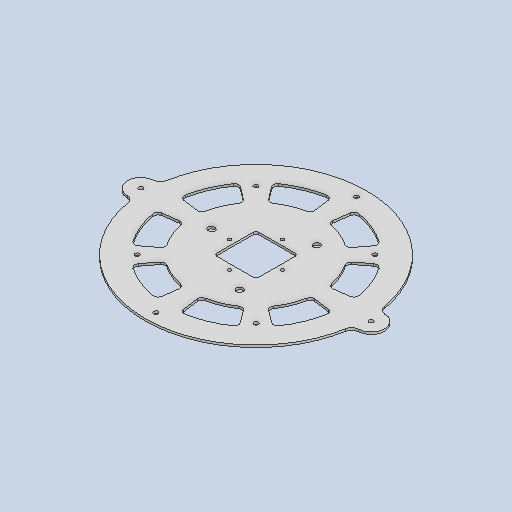
# Autodesk Inventor part: AP-1-02-basePlate
Saved by Autodesk Inventor 2025.1 (Build 291241020, 241B)
## iProperties
Created: 2024-10-16
Part Number: AP-1-02-basePlate
Material: Generic
Document SubType Name: Modeling
Designer: jdl5984
Density: 1 g/cm^3
Appearance: Default
Author: jdl5984
## iProperties of the stored document AP-1-02-basePlate_3DPrint.ipt
Created: 2024-12-05
Part Number: AP-1-02-basePlate_3DPrint
Material: Generic
Document SubType Name: Modeling
Designer: t205b
Density: 1 g/cm^3
Appearance: Default
Author: t205b
Autodesk Inventor part; units mm, degrees
ref_plane "YZ Plane" through (0, 0, 0) normal (1, 0, 0) x (0, 1, 0)
ref_plane "XZ Plane" through (0, 0, 0) normal (0, 1, 0) x (-1, 0, 0)
ref_plane "XY Plane" through (0, 0, 0) normal (0, 0, 1) x (1, 0, 0)
sketch "Sketch1" plane through (0, 0, 0) normal (0, 1, 0) x (-1, 0, 0)
  circle A0 centre (0, 0) radius 158.75
  line L0 (26.05, 30.05) -> (-26.05, 30.05)
  line L1 (-30.05, 26.05) -> (-30.05, -26.05)
  line L2 (-26.05, -30.05) -> (26.05, -30.05)
  line L3 (30.05, -26.05) -> (30.05, 26.05)
  arc A1 (30.05, 26.05) -> (26.05, 30.05) centre (26.05, 26.05) ccw
  arc A2 (26.05, -30.05) -> (30.05, -26.05) centre (26.05, -26.05) ccw
  arc A3 (-30.05, -26.05) -> (-26.05, -30.05) centre (-26.05, -26.05) ccw
  arc A4 (-26.05, 30.05) -> (-30.05, 26.05) centre (-26.05, 26.05) ccw
  circle A5 centre (38, 0) radius 2.5527
  circle A6 centre (0, -38) radius 2.5527
  circle A7 centre (-38, 0) radius 2.5527
  circle A8 centre (0, 38) radius 2.5527
  circle A9 centre (63.9092, 0) radius 4.7625
  circle A10 centre (-31.9546, -55.3454) radius 4.7625
  circle A11 centre (0, 0) radius 63.9092 construction
  circle A12 centre (0, 143.6497) radius 3.2067
  circle A13 centre (0, -143.6497) radius 3.2067
  line L4 (157.6029, 19.05) -> (165.227, 19.05)
  line L5 (165.227, 19.05) -> (165.227, -19.05) construction
  line L6 (165.227, -19.05) -> (157.6029, -19.05)
  line L7 (157.6029, -17.4578) -> (157.6029, 19.05) construction
  arc A14 (165.227, -19.05) -> (165.227, 19.05) centre (165.227, 0) ccw
  circle A15 centre (165.227, 0) radius 3.2067
  line L8 (0, -158.75) -> (0, 158.75) construction
  line L9 (-157.6029, 19.05) -> (-165.227, 19.05)
  line L10 (-165.227, -19.05) -> (-157.6029, -19.05)
  arc A16 (-165.227, 19.05) -> (-165.227, -19.05) centre (-165.227, 0) ccw
  circle A17 centre (-165.227, 0) radius 3.2067
  circle A18 centre (-31.9533, 55.3478) radius 4.7625
  point P0 (30.05, 30.05)
  point P1 (-30.05, 30.05)
  point P2 (30.05, -30.05)
  dimension "d0" = 317.5
  dimension "d1" = 30.05
  dimension "d2" = 60.1
  dimension "d3" = 60.1
  dimension "d4" = 30.05
  dimension "d5" = 4
  dimension "d6" = 4
  dimension "d7" = 5.1054
  dimension "d8" = 5.1054
  dimension "d9" = 5.1054
  dimension "d10" = 5.1054
  dimension "d11" = 76
  dimension "d12" = 38
  dimension "d13" = 76
  dimension "d14" = 38
  dimension "d15" = 9.525
  dimension "d17" = 110.6932
  dimension "d20" = 9.525
  dimension "d24" = 6.4135
  dimension "d25" = 6.4135
  dimension "d26" = 287.2994
  dimension "d27" = 143.6497
  dimension "d30" = 38.1
  dimension "d31" = 6.4135
  dimension "d33" = 330.454
  dimension "d38" = 110.6932
  dimension "d39" = 110.6932
  dimension "d41" = 127.8184
  constraints: 22 end point, 20 point on circle, 19 centre point, 8 tangent, 6 point on line, 6 symmetric about line, 4 coincident, 4 horizontal alignment, 4 parallel, 4 vertical alignment, 3 equal radius, 2 horizontal, 2 perpendicular, 1 midpoint, 1 vertical, 2 other
  measures "d0" diameter of A0
  measures "d1" distance from line of point (0, 0) L3
  measures "d2" distance of point (30.05, 30.05) point (-30.05, 30.05)
  measures "d3" distance of point (30.05, -30.05) point (30.05, 30.05)
  measures "d4" distance from line of point (0, 0) L2
  measures "d5" radius of A1
  measures "d6" radius of A2
  measures "d7" diameter of A5
  measures "d8" diameter of A6
  measures "d9" diameter of A7
  measures "d10" diameter of A8
  measures "d11" distance of A7.centre A5.centre
  measures "d12" distance of point (0, 0) A7.centre
  measures "d13" distance of A8.centre A6.centre
  measures "d14" distance of point (0, 0) A6.centre
  measures "d15" diameter of A9
  measures "d17" distance of A10.centre A9.centre
  measures "d20" diameter of A10
  measures "d24" diameter of A13
  measures "d25" diameter of A12
  measures "d26" distance of A13.centre A12.centre
  measures "d27" distance of A12.centre point (0, 0)
  measures "d30" distance of L4.start L6.end
  measures "d31" diameter of A15
  measures "d33" distance of A17.centre A14.centre
  measures "d38" distance of A18.centre A10.centre
  measures "d39" distance of A9.centre A18.centre
  measures "d41" diameter of A11
extrude "Extrusion1" add sketch "Sketch1" along normal blind 3.175
fillet "Fillet1" radius 10.16 4 edges at (-157.6029, 1.5875, 19.05) (-157.6029, 1.5875, -19.05) (157.6029, 1.5875, -19.05) (157.6029, 1.5875, 19.05)
sketch "Sketch4" plane through (0, 3.175, 0) normal (0, 1, 0) x (1, 0, 0)
  circle A0 centre (-85.3123, 85.3123) radius 3.175
  circle A1 centre (85.3122, 85.313) radius 3.175
  circle A2 centre (85.3123, -85.313) radius 3.175
  circle A3 centre (-85.3122, -85.3123) radius 3.175
  point P0 (0, 0)
  dimension "d79" = 6.35
  dimension "d80" = 6.35
  dimension "d81" = 6.35
  dimension "d82" = 6.35
  dimension "d83" = 241.3
  dimension "d84" = 170.6245
  dimension "d85" = 170.6245
  dimension "d86" = 241.3
  dimension "d94" = 85.3123
  dimension "d95" = 85.3123
  constraints: 4 centre point, 2 vertical alignment
  measures "d79" diameter of A0
  measures "d80" diameter of A1
  measures "d81" diameter of A2
  measures "d82" diameter of A3
  measures "d83" distance of A2.centre A0.centre
  measures "d84" distance of A3.centre A0.centre
  measures "d85" distance of A1.centre A0.centre
  measures "d86" distance of A3.centre A1.centre
  measures "d94" horizontal distance of A2.centre point (0, 0)
  measures "d95" horizontal distance of point (0, 0) A3.centre
extrude "Extrusion3" cut sketch "Sketch4" against normal blind 6.35
sketch "Sketch2" plane through (0, 3.175, 0) normal (0, 1, 0) x (1, 0, 0)
  circle A0 centre (0, 0) radius 127
  circle A1 centre (0, 0) radius 92.075
  line L0 (-56.0517, 73.048) -> (-77.3127, 100.7559)
  line L1 (-73.048, 56.0517) -> (-100.7559, 77.3127)
  line L2 (0, -163.1298) -> (0, 179.0381) construction
  line L3 (-207.243, 0) -> (231.1977, 0) construction
  arc A2 (156.3619, 27.432) -> (-156.3619, 27.432) centre (0, 0) ccw projected
  line L4 (-91.2873, 12.0182) -> (-125.9135, 16.5768)
  line L5 (-91.2873, -12.0182) -> (-125.9135, -16.5768)
  line L6 (-73.048, -56.0517) -> (-100.7559, -77.3127)
  line L7 (-56.0517, -73.048) -> (-77.3127, -100.7559)
  line L8 (-12.0182, -91.2873) -> (-16.5768, -125.9135)
  line L9 (12.0182, -91.2873) -> (16.5768, -125.9135)
  line L10 (56.0517, -73.048) -> (77.3127, -100.7559)
  line L11 (73.048, -56.0517) -> (100.7559, -77.3127)
  line L12 (91.2873, -12.0182) -> (125.9135, -16.5768)
  line L13 (91.2873, 12.0182) -> (125.9135, 16.5768)
  line L14 (73.048, 56.0517) -> (100.7559, 77.3127)
  line L15 (56.0517, 73.048) -> (77.3127, 100.7559)
  line L16 (12.0182, 91.2873) -> (16.5768, 125.9135)
  line L17 (-12.0182, 91.2873) -> (-16.5768, 125.9135)
  dimension "d96" = 254
  dimension "d97" = 184.15
  dimension "d98" = 15
  dimension "d99" = 37.5
  dimension "d102" = 360
  constraints: 36 end point, 4 line through centre, 4 point on circle, 2 centre point, 2 coincident, 1 concentric, 1 horizontal, 1 vertical, 49 other
  measures "d96" diameter of A0
  measures "d97" diameter of A1
  measures "d98" angle of L1 L0
  measures "d99" angle of L2 L0
extrude "Extrusion2" cut sketch "Sketch2" against normal blind 6.35 contours L13 A1 L14 A0 | A0 L11 A1 L12 | L15 A1 L16 A0 | A0 L9 A1 L10 | L17 A1 L0 A0 | A0 L7 A1 L8 | L1 A1 L4 A0 | A0 L5 A1 L6
fillet "Fillet5" radius 6.35 32 edges at (77.3127, 1.5875, -100.7559) (100.7559, 1.5875, -77.3127) (73.048, 1.5875, -56.0517) (56.0517, 1.5875, -73.048) (91.2873, 1.5875, -12.0182) (125.9135, 1.5875, -16.5768) (125.9135, 1.5875, 16.5768) (91.2873, 1.5875, 12.0182) (100.7559, 1.5875, 77.3127) (73.048, 1.5875, 56.0517) (56.0517, 1.5875, 73.048) (12.0182, 1.5875, 91.2873) (16.5768, 1.5875, 125.9135) (77.3127, 1.5875, 100.7559) (-16.5768, 1.5875, 125.9135) (-12.0182, 1.5875, 91.2873) (-56.0517, 1.5875, 73.048) (-77.3127, 1.5875, 100.7559) (-100.7559, 1.5875, 77.3127) (-73.048, 1.5875, 56.0517) (-91.2873, 1.5875, 12.0182) (-125.9135, 1.5875, 16.5768) (-91.2873, 1.5875, -12.0182) (-125.9135, 1.5875, -16.5768) (-100.7559, 1.5875, -77.3127) (-73.048, 1.5875, -56.0517) (16.5768, 1.5875, -125.9135) (12.0182, 1.5875, -91.2873) (-12.0182, 1.5875, -91.2873) (-16.5768, 1.5875, -125.9135) (-77.3127, 1.5875, -100.7559) (-56.0517, 1.5875, -73.048)
sketch "Sketch5" plane through (0, 3.175, 0) normal (0, 1, 0) x (1, 0, 0)
  arc A0 (156.3619, 27.432) -> (-156.3619, 27.432) centre (0, 0) ccw projected
  line L0 (114.3236, 93.5033) -> (107.7468, 85.6097)
  line L1 (102.7949, 85.7011) -> (98.9428, 90.6878)
  line L2 (96.4302, 91.9218) -> (82.6421, 91.9218)
  line L3 (79.821, 90.2034) -> (62.9267, 57.4822)
  line L4 (58.0732, 56.4995) -> (54.345, 59.6057)
  line L5 (49.5395, 58.7126) -> (43.6449, 48.1401)
  line L6 (45.7335, 43.4937) -> (54.672, 41.52)
  line L7 (55.9284, 35.907) -> (38.3968, 22.3645)
  line L8 (36.4558, 21.7021) -> (30.05, 21.7021)
  arc A1 (114.3236, 93.5033) -> (114.0851, 97.8242) centre (111.8843, 95.5356) ccw
  arc A2 (102.7949, 85.7011) -> (107.7468, 85.6097) centre (105.3075, 87.642) ccw
  arc A3 (98.9428, 90.6878) -> (96.4302, 91.9218) centre (96.4302, 88.7468) ccw
  arc A4 (82.6421, 91.9218) -> (79.821, 90.2034) centre (82.6421, 88.7468) ccw
  arc A5 (58.0732, 56.4995) -> (62.9267, 57.4822) centre (60.1056, 58.9387) ccw
  arc A6 (54.345, 59.6057) -> (49.5395, 58.7126) centre (52.3126, 57.1665) ccw
  arc A7 (43.6449, 48.1401) -> (45.7335, 43.4937) centre (46.418, 46.594) ccw
  arc A8 (55.9284, 35.907) -> (54.672, 41.52) centre (53.9875, 38.4197) ccw
  arc A9 (36.4558, 21.7021) -> (38.3968, 22.3645) centre (36.4558, 24.8771) ccw
  line L9 (30.05, 26.05) -> (30.05, -26.05) projected
  line L10 (-117.6843, 106.5457) -> (-111.6904, 95.8778)
  line L11 (-117.6843, 106.5457) -> (-105.4478, 106.5457) construction
  line L12 (-106.3149, 95.6214) -> (-100.0956, 104.573)
  line L13 (-95.2104, 104.9733) -> (-73.8025, 82.9275)
  line L14 (-74.5251, 77.9476) -> (-78.9198, 75.4784)
  line L15 (-78.6641, 69.8135) -> (-51.9607, 57.8342)
  line L16 (-47.4862, 60.7311) -> (-47.4862, 61.3366)
  line L17 (-44.7451, 64.4818) -> (-25.6966, 67.1097)
  line L18 (-22.1466, 64.5733) -> (-15.4011, 30.05)
  line L19 (-26.05, 30.05) -> (26.05, 30.05) projected
  arc A10 (-111.6904, 95.8778) -> (-106.3149, 95.6214) centre (-108.9224, 97.433) ccw
  arc A11 (-95.2104, 104.9733) -> (-100.0956, 104.573) centre (-97.4881, 102.7614) ccw
  arc A12 (-74.5251, 77.9476) -> (-73.8025, 82.9275) centre (-76.0803, 80.7156) ccw
  arc A13 (-78.9198, 75.4784) -> (-78.6641, 69.8135) centre (-77.3645, 72.7104) ccw
  arc A14 (-51.9607, 57.8342) -> (-47.4862, 60.7311) centre (-50.6612, 60.7311) ccw
  arc A15 (-22.1466, 64.5733) -> (-25.6966, 67.1097) centre (-25.2627, 63.9644) ccw
  arc A16 (-44.7451, 64.4818) -> (-47.4862, 61.3366) centre (-44.3112, 61.3366) ccw
  arc A17 (-156.3619, -27.432) -> (156.3619, -27.432) centre (0, 0) ccw projected
  line L20 (119.7564, -104.2111) -> (114.1977, -94.483)
  line L21 (109.9208, -93.2708) -> (97.3336, -100.1357)
  line L22 (93.7922, -99.7968) -> (75.1242, -84.3868)
  line L23 (76.2302, -78.898) -> (76.7833, -78.7315)
  line L24 (76.89, -72.6852) -> (51.4176, -64.0266)
  line L25 (49.6689, -59.4699) -> (57.6248, -45.2546)
  line L26 (53.334, -40.9166) -> (42.263, -46.9545)
  line L27 (39.9931, -47.2523) -> (30.8267, -45.025)
  line L28 (29.5587, -33.3702) -> (19.9311, -30.05)
  line L29 (26.05, -30.05) -> (-26.05, -30.05) projected
  arc A18 (30.05, -39.1557) -> (29.5587, -33.3702) centre (28.5236, -36.3717) ccw
  arc A19 (30.05, -39.1557) -> (30.8267, -45.025) centre (31.5764, -41.9397) ccw
  arc A20 (39.9931, -47.2523) -> (42.263, -46.9545) centre (40.7428, -44.1671) ccw
  arc A21 (57.6248, -45.2546) -> (53.334, -40.9166) centre (54.8542, -43.704) ccw
  arc A22 (49.6689, -59.4699) -> (51.4176, -64.0266) centre (52.4395, -61.0205) ccw
  arc A23 (76.7833, -78.7315) -> (76.89, -72.6852) centre (75.8682, -75.6913) ccw
  arc A24 (76.2302, -78.898) -> (75.1242, -84.3868) centre (77.1454, -81.9382) ccw
  arc A25 (93.7922, -99.7968) -> (97.3336, -100.1357) centre (95.8134, -97.3483) ccw
  arc A26 (114.1977, -94.483) -> (109.9208, -93.2708) centre (111.441, -96.0582) ccw
  line L30 (-104.9788, -99.3397) -> (-112.1614, -95.7578)
  line L31 (-112.2322, -90.1116) -> (-82.8881, -74.5468)
  line L32 (-78.3749, -76.3889) -> (-76.3512, -82.7485)
  line L33 (-70.1534, -81.9173) -> (-68.7033, -46.9526)
  line L34 (-68.7909, -46.069) -> (-70.602, -38.6403)
  line L35 (-66.8156, -34.7917) -> (-52.1965, -38.1049)
  line L36 (-48.4101, -34.2563) -> (-51.9142, -19.8837)
  line L37 (-50.1979, -16.2666) -> (-30.05, -6.6439)
  line L38 (-30.05, -26.05) -> (-30.05, 26.05) projected
  arc A27 (-50.1979, -16.2666) -> (-51.9142, -19.8837) centre (-48.8295, -19.1316) ccw
  arc A28 (-52.1965, -38.1049) -> (-48.4101, -34.2563) centre (-51.4947, -35.0084) ccw
  arc A29 (-66.8156, -34.7917) -> (-70.602, -38.6403) centre (-67.5174, -37.8882) ccw
  arc A30 (-68.7033, -46.9526) -> (-68.7909, -46.069) centre (-71.8755, -46.821) ccw
  arc A31 (-76.3512, -82.7485) -> (-70.1534, -81.9173) centre (-73.3257, -81.7857) ccw
  arc A32 (-78.3749, -76.3889) -> (-82.8881, -74.5468) centre (-81.4004, -77.3517) ccw
  arc A33 (-112.2322, -90.1116) -> (-112.1614, -95.7578) centre (-110.7444, -92.9165) ccw
  arc A34 (-106.0677, -105.339) -> (-104.9788, -99.3397) centre (-106.3957, -102.181) ccw
  line L39 (-106.0677, -105.339) -> (-117.6843, -106.5457)
  line L40 (-15.4011, 30.05) -> (-30.05, -6.6439)
  line L41 (30.05, 21.7021) -> (19.9311, -30.05)
  arc A35 (113.1683, 100.7146) -> (114.0851, 97.8242) centre (116.2858, 100.1127) ccw
  line L42 (113.1683, 100.7146) -> (114.8773, 109.5663)
  point P0 (-30.05, -6.6439)
  point P1 (-59.506, -36.4483)
  point P2 (-65.3124, 63.8239)
  dimension "d107" = 3.175
  dimension "d108" = 3.175
  dimension "d109" = 3.175
  dimension "d119" = 11.6166
  dimension "d120" = 10.5725
  dimension "d121" = 8.9385
  dimension "d122" = 16.8942
  dimension "d123" = 9.6276
  dimension "d124" = 5.5587
  dimension "d125" = 9.7281
  dimension "d126" = 18.668
  dimension "d127" = 13.5426
  dimension "d128" = 6.4058
  dimension "d129" = 8.3479
  dimension "d130" = 0.5531
  dimension "d131" = 3.175
  dimension "d132" = 8.8517
  dimension "d133" = 1.9736
  constraints: 78 end point, 74 point on circle, 65 tangent, 34 centre point, 30 equal radius, 8 point on line, 3 horizontal, 3 parallel, 3 perpendicular, 2 midpoint, 1 equal length, 1 vertical, 28 other
  measures "d107" radius of A10
  measures "d108" radius of A18
  measures "d109" radius of A27
  measures "d119" horizontal distance of L39.start L39.end
  measures "d120" vertical distance of L5.start L5.end
  measures "d121" horizontal distance of L6.start L6.end
  measures "d122" horizontal distance of L3.start L3.end
  measures "d123" horizontal distance of L28.start L28.end
  measures "d124" horizontal distance of L20.start L20.end
  measures "d125" vertical distance of L20.start L20.end
  measures "d126" horizontal distance of L22.start L22.end
  measures "d127" vertical distance of L7.start L7.end
  measures "d128" distance of L8.start L8.end
  measures "d129" distance between parallel lines of L19 L8
  measures "d130" horizontal distance of L23.start L23.end
  measures "d131" radius of A35
  measures "d132" vertical distance of L42.start L42.end
  measures "d133" vertical distance of L6.start L6.end
split "Split17" [suppressed]
split "Split18" [suppressed]
sketch "Sketch6" plane through (0, 3.175, 0) normal (0, 1, 0) x (1, 0, 0)
  line L0 (26.7247, 0) -> (-26.85, 0)
  line L1 (-30.05, -6.6439) -> (-30.05, 26.05) projected
  point P0 (0, 0)
  constraints: 2 end point, 1 perpendicular
split "Split19" [suppressed]
equation "\"d24\" = d25"
equation "\"d25\" = d31"
equation "\"d38\" = d17"
equation "\"d39\" = d17"
body "Solid1"
body "Solid34"
body "Solid35"
body "Solid38"
body "Solid39"
body "Solid40"
body "Solid41"
